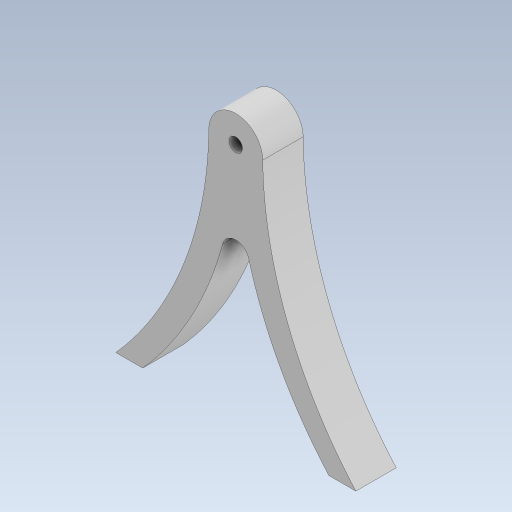
# Autodesk Inventor part: transfer gear rod support
Saved by Autodesk Inventor 2023 (Build 270158000, 158)
## iProperties
Created: 2023-03-23
Part Number: transfer gear rod support
Material: Generic
Document SubType Name: Modeling
Designer: dverd
Density: 1 g/cm^3
Appearance: Default
Author: dverd
Autodesk Inventor part; units mm, degrees
ref_plane "XZ Plane" through (0, 0, 0) normal (0, 1, 0) x (-1, 0, 0)
ref_plane "XY Plane" through (0, 0, 0) normal (0, 0, 1) x (1, 0, 0)
sketch "Sketch1" plane through (0, 0, 0) normal (0, 0, 1) x (1, 0, 0)
  line L0 (0, 0) -> (56.6166, 0)
  line L1 (56.6166, 0) -> (56.6166, 56.6166)
  line L2 (56.6166, 56.6166) -> (0, 56.6166)
  line L3 (0, 56.6166) -> (0, 0)
  circle A0 centre (28.3083, 56.6166) radius 1.5635
  circle A1 centre (28.3083, 56.6166) radius 6.35
  arc A2 (0, 0) -> (21.9587, 56.6898) centre (-64.7797, 57.6901) ccw
  arc A3 (6.3496, 0) -> (25.2456, 34.8225) centre (-58.4301, 57.6901) ccw
  line L4 (28.3083, 0) -> (28.3083, 56.6898)
  arc A4 (34.6579, 56.6898) -> (56.6166, 0) centre (121.3963, 57.6901) ccw
  arc A5 (31.371, 34.8225) -> (50.267, 0) centre (115.0467, 57.6901) ccw
  arc A6 (31.371, 34.8225) -> (25.2456, 34.8225) centre (28.3083, 33.9855) ccw
  point P0 (21.9583, 56.6166)
  point P1 (21.9578, 56.6166)
  point P2 (6.3496, 0)
  point P3 (50.267, 0)
  point P4 (34.6588, 56.6166)
  point P5 (34.6583, 56.6166)
  dimension "d3" = 12.7
  dimension "d0" = 56.6166
  dimension "d1" = 56.6166
  dimension "d2" = 3.127
  dimension "d4" = 3.175
  constraints: 12 point on circle, 10 end point, 6 centre point, 4 symmetric about line, 2 midpoint, 2 parallel, 2 tangent, 1 coincident, 1 horizontal, 1 perpendicular, 1 vertical, 6 other
  measures "d0" distance of L2.end L1.end
  measures "d1" distance of L1.end L0.end
  measures "d2" diameter of A0
  measures "d4" radius of A6
extrude "Extrusion1" add sketch "Sketch1" along normal blind 9.525 contours A2 A1 L4 A6 A3 L0 | A1 L2 A0 | L2 A0 L4 A1 | L4 A0 L2 A1 | A1 A4 L0 A5 A6 L4
ref_plane "Work Plane2" through (28.3083, 0, 0) normal (1, 0, 0) x (0, 1, 0)
ref_plane "Work Plane1" through (56.6166, 0, 0) normal (1, 0, 0) x (0, 1, 0)
body "Solid1"
